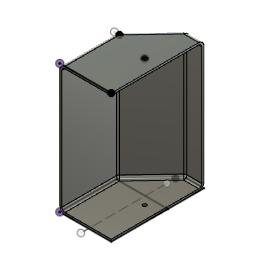
toolbox-top (Autodesk Fusion 360 design; units mm, degrees)
Autodesk Fusion 360 part; units mm, degrees
sketch "Sketch1" plane through (0, 0, 0) normal (0, 1, 0) x (1, 0, 0)
  line L0 (0, 0) -> (50, 0)
  line L1 (50, 0) -> (50, 55)
  line L2 (50, 55) -> (0, 55)
  line L3 (0, 55) -> (0, 0)
  line L4 (50, 55) -> (50, 90)
  line L5 (50, 90) -> (33.3333, 90)
  line L6 (33.3333, 90) -> (0, 55)
  line L7 (28, 76) -> (28, -7.4569) construction
  point P0 (28, 84.4)
  dimension "d1" = 50
  dimension "d2" = 55
  dimension "d3" = 35
  dimension "d4" = 16.6667
  dimension "d17" = 22
  constraint horizontal L0
  constraint vertical L1
  constraint horizontal L2
  constraint vertical L3
  constraint coincident L0.start L3.end
  constraint perpendicular L2 L4
  constraint perpendicular L1 L5
  constraint vertical L7
  constraint coincident L6 P0
  constraint coincident L7 P0
  measures "d1" distance of L0.start L0.end
  measures "d2" distance of L0.start L2.end
  measures "d3" distance of L1.end L4.end
  measures "d4" distance of L4.end L5.end
  measures "d17" distance of L1 L7
extrude "Extrude1" add sketch "Sketch1" along normal blind 125
fillet "Fillet1" radius 5 1 edges at (0, 125, -27.5)
fillet "Fillet2" radius 5 1 edges at (0, 0, -27.5)
fillet "Fillet3" radius 5 7 edges at (19.1667, 125, -75.125) (1.4645, 123.5355, -56.5377) (0, 62.5, -55) (1.4645, 1.4645, -56.5377) (19.1667, 0, -75.125) (41.6667, 125, -90) (41.6667, 0, -90)
fillet "Fillet4" radius 5 3 edges at (33.961, 1.4645, -88.5355) (33.3333, 62.5, -90) (33.961, 123.5355, -88.5355)
shell "Shell1" thickness 2 removed faces 2 at (50, 43.3333, -30) at (33.3333, 81.6667, 0)
sketch "Sketch2" plane through (0, 125, 0) normal (0, 1, 0) x (-1, 0, 0)
  line L0 (-50, -85) -> (-35.4762, -85)
  line L1 (-35.4762, -85) -> (-5, -53)
  line L2 (-5, -53) -> (-5, 0)
  line L3 (-5, 0) -> (-50, 0)
  line L4 (-50, 0) -> (-50, -85)
  line L5 (0, 0) -> (-50, 0)
  line L6 (-5, -53) -> (0, -53)
  circle A0 centre (-37.5, -45) radius 1.75
  dimension "d12" = 3.5
  dimension "d13" = 12.5
  dimension "d16" = 45
  constraint coincident L5.start origin
  constraint coincident L3.end L4.start
  constraint coincident L1.end L2.start
  constraint perpendicular L2 L6
  measures "d12" diameter of A0
  measures "d13" distance of L4 A0.centre
  measures "d16" distance of L5 A0.centre
extrude "Extrude2" cut sketch "Sketch2" against normal up to surface (125 mm away) contours A0
equation "d4 = d1 / 3"
